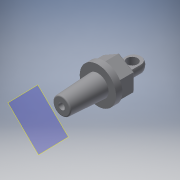
# Autodesk Inventor part: cast1
Saved by Autodesk Inventor 2016 (Build 200138000, 138)
## iProperties
Created: 2016-11-29
Part Number: cast1
Material: Generic
Document SubType Name: Modeling
Designer: Juraj
Density: 1 g/cm^3
Appearance: Default
Author: Juraj
Autodesk Inventor part; units mm, degrees
ref_plane "YZ Plane" through (0, 0, 0) normal (1, 0, 0) x (0, 1, 0)
ref_plane "XZ Plane" through (0, 0, 0) normal (0, 1, 0) x (-1, 0, 0)
ref_plane "XY Plane" through (0, 0, 0) normal (0, 0, 1) x (1, 0, 0)
sketch "Sketch1" plane through (0, 0, 0) normal (0, 1, 0) x (-1, 0, 0)
  circle A0 centre (0, 0) radius 8.5
  dimension "d0" = 17
  constraints: 1 centre point, 1 coincident
  measures "d0" diameter of A0
extrude "Extrusion1" add sketch "Sketch1" along normal blind 3
sketch "Sketch2" plane through (0, 3, 0) normal (0, 1, 0) x (1, 0, 0)
  line L0 (-7.0206, 4.0055) -> (-0.0415, 8.0828)
  line L1 (-0.0415, 8.0828) -> (6.9792, 4.0773)
  line L2 (6.9792, 4.0773) -> (7.0206, -4.0055)
  line L3 (7.0206, -4.0055) -> (0.0415, -8.0828)
  line L4 (0.0415, -8.0828) -> (-6.9792, -4.0773)
  line L5 (-6.9792, -4.0773) -> (-7.0206, 4.0055)
  point P0 (0, 0)
  point P1 (0, 0)
  dimension "d3" = 14
  constraints: 12 end point, 1 coincident, 13 other
  measures "d3" distance between parallel lines of L2 L5
extrude "Extrusion2" add sketch "Sketch2" along normal blind 7
fillet "Fillet1" radius 0.5 6 edges at (3.531, 10, 6.0441) (6.9999, 10, -0.0359) (-3.4689, 10, 6.08) (-6.9999, 10, 0.0359) (-3.531, 10, -6.0441) (3.4689, 10, -6.08)
sketch "Sketch3" plane through (0, 10, 0) normal (0, 1, 0) x (1, 0, 0)
  circle A0 centre (0, 0) radius 3.85
  dimension "d7" = 7.7
  constraints: 1 centre point, 1 coincident
  measures "d7" diameter of A0
extrude "Extrusion3" add sketch "Sketch3" along normal blind 0.8
sketch "Sketch4" plane through (0, 10.8, 0) normal (0, 1, 0) x (1, 0, 0)
  circle A0 centre (0, 0) radius 3.85 projected
  line L0 (-3.4033, -1.8) -> (3.4033, -1.8)
  line L1 (-3.4033, 1.8) -> (3.4033, 1.8)
  arc A1 (-3.4033, 1.8) -> (-3.4033, -1.8) centre (0, 0) ccw
  arc A2 (3.4033, -1.8) -> (3.4033, 1.8) centre (0, 0) ccw
  dimension "d11" = 3.6
  constraints: 8 point on circle, 4 end point, 2 centre point, 1 concentric
  measures "d11" distance between parallel lines of L1 L0
extrude "Extrusion4" add sketch "Sketch4" along normal blind 9.8 contours A0 L0 L1
sketch "Sketch5" plane through (-3.4033, 10.8, 1.8) normal (0, 0, 1) x (1, 0, 0)
  circle A0 centre (3.4, 5.3) radius 2.5
  line L0 (0, 0) -> (0, 9.8) projected
  line L1 (6.8066, 0) -> (6.8066, 9.8) projected
  line L2 (0, 9.8) -> (6.8066, 9.8) projected
  point P0 (3.4033, -10.8)
  dimension "d15" = 5
  dimension "d16" = 3.4
  dimension "d17" = 3.4066
  dimension "d18" = 4.5
  constraints: 1 centre point
  measures "d15" diameter of A0
  measures "d16" distance from line of A0.centre L0
  measures "d17" distance from line of L1 A0.centre
  measures "d18" distance from line of L2 A0.centre
extrude "Extrusion5" cut sketch "Sketch5" against normal blind 9.8
fillet "Fillet3" radius 3.85 1 edges at (3.85, 20.6, 0)
sketch "Sketch6" plane through (0, 0, 0) normal (0, -1, 0) x (1, 0, 0)
  circle A0 centre (0, 0) radius 5
  dimension "d22" = 10
  constraints: 1 centre point, 1 coincident
  measures "d22" diameter of A0
extrude "Extrusion6" add sketch "Sketch6" along normal blind 17
draft "FaceDraft1" angle 3 pull direction (0, -1, 0) faces at (4.9353, -11.3333, -0.8021) fixed edges at (-5, 0, 0)
sketch "Sketch8" plane through (0, -17, 0) normal (0, -1, 0) x (1, 0, 0)
  circle A0 centre (0, 0) radius 1.5
  dimension "d26" = 3
  constraints: 1 centre point, 1 coincident
  measures "d26" diameter of A0
extrude "Extrusion7" cut sketch "Sketch8" against normal blind 15
fillet "Fillet4" radius 0.3 2 edges at (0, 10.8, 3.85) (0, 10.8, -3.85)
ref_plane "Work Plane1" through (0, -28, 0) normal (0, 1, 0) x (0.6995635, 0, 0.7145704)
fillet "Fillet5" radius 0.6 1 edges at (-4.1091, -17, 0)
body "Solid1"
